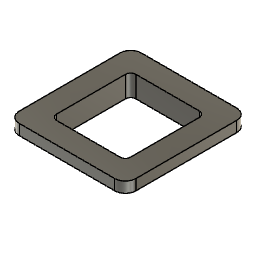
frames (Autodesk Fusion 360 design; units mm, degrees)
Autodesk Fusion 360 part; units mm, degrees
sketch "Esboço1" plane through (0, 0, 0) normal (0, 0, 1) x (1, 0, 0)
  line L0 (9, 9.5) -> (-9, 9.5)
  line L1 (-9, 9.5) -> (-9, -9.5)
  line L2 (-9, -9.5) -> (9, -9.5)
  line L3 (9, -9.5) -> (9, 9.5)
  line L4 (9, 9.5) -> (-9, -9.5) construction
  line L5 (-9, 9.5) -> (9, -9.5) construction
  line L6 (-7, -7.5) -> (7, -7.5)
  line L7 (7, -7.5) -> (7, 7.5)
  line L8 (7, 7.5) -> (-7, 7.5)
  line L9 (-7, 7.5) -> (-7, -7.5)
  dimension "d1" = 18
  dimension "d2" = 19
  dimension "d3" = -2
  constraint horizontal L0
  constraint perpendicular L0 L1
  constraint parallel L0 L2
  constraint parallel L1 L3
  constraint coincident L4 origin
  constraint coincident L5 origin
  measures "d1" distance of L1.end L2.end
  measures "d2" distance of L0.end L1.end
extrude "Extrusão1" add sketch "Esboço1" along normal blind 2
sketch "Esboço2" plane through (0, 0, 2) normal (0, 0, 1) x (-1, 0, 0)
  line L0 (7, 7.5) -> (7, -7.5)
  line L1 (7, -7.5) -> (-7, -7.5)
  line L2 (-7, -7.5) -> (-7, 7.5)
  line L3 (-7, 7.5) -> (7, 7.5)
  line L4 (-9, 9.5) -> (-9, -9.5)
  line L5 (-9, -9.5) -> (9, -9.5)
  line L6 (9, -9.5) -> (9, 9.5)
  line L7 (9, 9.5) -> (-9, 9.5)
  line L8 (-11, 9.5) -> (-11, -9.5)
  line L9 (-9, -11.5) -> (9, -11.5)
  line L10 (11, -9.5) -> (11, 9.5)
  line L11 (9, 11.5) -> (-9, 11.5)
  arc A0 (11, 9.5) -> (9, 11.5) centre (9, 9.5) ccw
  arc A1 (-9, 11.5) -> (-11, 9.5) centre (-9, 9.5) ccw
  arc A2 (-11, -9.5) -> (-9, -11.5) centre (-9, -9.5) ccw
  arc A3 (9, -11.5) -> (11, -9.5) centre (9, -9.5) ccw
  dimension "d7" = 2
  constraint tangent L10 A0
  constraint tangent L11 A0
  constraint tangent L11 A1
  constraint tangent L8 A1
  constraint equal A0 A1
  constraint tangent L8 A2
  constraint tangent L9 A2
  constraint equal A0 A2
  constraint tangent L10 A3
  constraint tangent L9 A3
  constraint equal A0 A3
  measures "d7" radius of A0
extrude "Extrusão2" add sketch "Esboço2" along normal blind 2 contours L4 L5 L6 L7 | L8 L9 L10 L11 A0 A1 A2 A3
fillet "Arredondamento1" radius 2 4 edges at (-9, 9.5, 1) (-9, -9.5, 1) (9, 9.5, 1) (9, -9.5, 1)
fillet "Arredondamento2" radius 1 4 edges at (-7, 7.5, 2) (-7, -7.5, 2) (7, -7.5, 2) (7, 7.5, 2)
